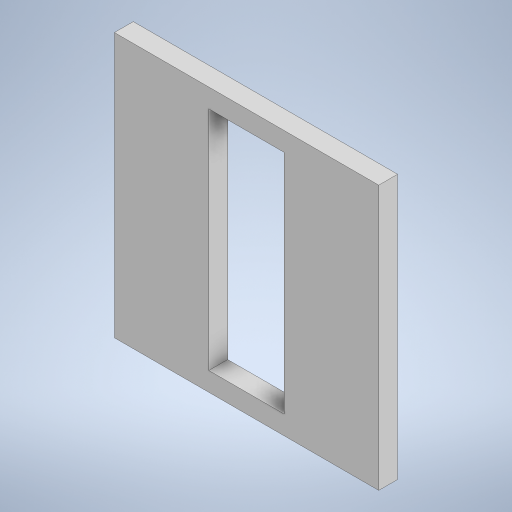
# Autodesk Inventor part: JukeBox Top Panel SQ
Saved by Autodesk Inventor 2024 (Build 280153000, 153)
## iProperties
Created: 2023-04-22
Part Number: JukeBox Top Panel SQ
Material: Generic
Document SubType Name: Modeling
Designer: newic
Density: 1 g/cm^3
Appearance: Default
Author: newic
Autodesk Inventor part; units mm, degrees
ref_plane "YZ Plane" through (0, 0, 0) normal (1, 0, 0) x (0, 1, 0)
ref_plane "XZ Plane" through (0, 0, 0) normal (0, 1, 0) x (-1, 0, 0)
ref_plane "XY Plane" through (0, 0, 0) normal (0, 0, 1) x (1, 0, 0)
sketch "Sketch1" plane through (0, 0, 0) normal (0, 0, 1) x (1, 0, 0)
  line L0 (0, 0) -> (812.8, 0) construction
  line L1 (812.8, 0) -> (812.8, -406.4) construction
  line L2 (812.8, -406.4) -> (0, -406.4) construction
  line L3 (0, -406.4) -> (0, 0) construction
  line L4 (0, 0) -> (406.4, 0)
  line L5 (406.4, 0) -> (406.4, -25.4)
  line L6 (406.4, -25.4) -> (0, -25.4)
  line L7 (0, -25.4) -> (0, 0)
  line L8 (406.4, -25.4) -> (381, -25.4)
  line L9 (381, -25.4) -> (381, -406.4)
  line L10 (381, -406.4) -> (406.4, -406.4)
  line L11 (406.4, -406.4) -> (406.4, -25.4)
  line L12 (381, -406.4) -> (0, -406.4)
  line L13 (0, -406.4) -> (0, -381)
  line L14 (0, -381) -> (381, -381)
  line L15 (381, -381) -> (381, -406.4)
  line L16 (0, -381) -> (25.4, -381)
  line L17 (25.4, -381) -> (25.4, -25.4)
  line L18 (25.4, -25.4) -> (0, -25.4)
  line L19 (0, -25.4) -> (0, -381)
  dimension "d1" = 812.8
  dimension "d5" = 406.4
  dimension "d6" = 25.4
  dimension "d7" = 25.4
  dimension "d8" = 381
  dimension "d9" = 381
  dimension "d10" = 25.4
  dimension "d11" = 25.4
  constraints: 32 end point, 8 parallel, 4 horizontal, 4 perpendicular, 1 point on line, 2 other
  measures "d1" distance of L1.end L2.end
  measures "d5" distance of L5.end L6.end
  measures "d6" distance of L4.end L5.end
  measures "d7" distance of L10.end L9.end
  measures "d8" distance of L9.end L8.end
  measures "d9" distance of L13.end L14.end
  measures "d10" distance of L12.end L13.end
  measures "d11" distance of L18.end L17.end
extrude "Extrusion1" add sketch "Sketch1" against normal blind 25.4 contours L6 L9 L14 L17
sketch "Sketch3" plane through (0, 0, 0) normal (0, 0, 1) x (1, 0, 0)
  line L0 (-406.4, 0) -> (406.4, 0) construction
  line L1 (406.4, 0) -> (406.4, -406.4) construction
  line L2 (406.4, -406.4) -> (-406.4, -406.4) construction
  line L3 (-406.4, -406.4) -> (-406.4, 0) construction
  line L4 (406.4, 0) -> (406.4, -406.4)
  line L5 (381, -381) -> (25.4, -381) projected
  line L6 (203.2, -381) -> (203.2, -355.6)
  line L7 (203.2, -355.6) -> (254, -355.6)
  line L8 (254, -355.6) -> (254, -50.8)
  line L9 (254, -50.8) -> (152.4, -50.8)
  line L10 (152.4, -50.8) -> (152.4, -355.6)
  line L11 (152.4, -355.6) -> (203.2, -355.6)
  point P0 (0, 0)
  dimension "d36" = 812.8
  dimension "d45" = 25.4
  dimension "d46" = 50.8
  dimension "d47" = 304.8
  dimension "d48" = 101.6
  constraints: 16 end point, 4 perpendicular, 1 collinear, 1 midpoint, 1 point on line, 1 vertical, 2 other
  measures "d36" distance of L1.end L2.end
  measures "d45" distance of L6.start L6.end
  measures "d46" distance of L6.end L7.end
  measures "d47" distance of L7.end L8.end
  measures "d48" distance of L8.end L9.end
extrude "Extrusion3" cut sketch "Sketch3" against normal blind 25.4
body "Solid1"
